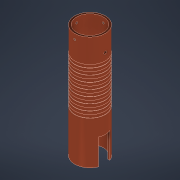
# Autodesk Inventor part: Test_Radiator
Saved by Autodesk Inventor 2022 (Build 260153000, 153)
## iProperties
Created: 2024-05-08
Part Number: Test_Radiator
Material: Generic
Document SubType Name: Modeling
Designer: jo_ki
Density: 1 g/cm^3
Appearance: Copper - Polished
Mass: 36.3453 g
Surface Area: 313.53 cm^2
Volume: 36.3453 cm^3
Author: jo_ki
Autodesk Inventor part; units mm, degrees
note: some values were not read from the file. Chosen so that the rebuilt part matches the saved one: pattern direction of "Circular Pattern1".
ref_plane "XZ Plane" through (0, 0, 0) normal (0, 1, 0) x (-1, 0, 0)
sketch "Sketch1" plane through (0, 0, 0) normal (0, 0, 1) x (1, 0, 0)
  line L0 (0, -89.875) -> (0, 76.375) projected
  line L1 (0, 24.375) -> (14, 24.375)
  line L2 (14, 24.375) -> (14, 21.125)
  line L3 (14, 21.125) -> (20, 21.125)
  line L4 (20, 21.125) -> (20, 17.875)
  line L5 (20, 17.875) -> (14, 17.875)
  line L6 (14, 17.875) -> (14, 14.625)
  line L7 (14, 14.625) -> (20, 14.625)
  line L8 (20, 14.625) -> (20, 11.375)
  line L9 (20, 11.375) -> (14, 11.375)
  line L10 (14, 11.375) -> (14, 8.125)
  line L11 (14, 8.125) -> (20, 8.125)
  line L12 (20, 8.125) -> (20, 4.875)
  line L13 (20, 4.875) -> (14, 4.875)
  line L14 (14, 4.875) -> (14, 1.625)
  line L15 (14, 1.625) -> (20, 1.625)
  line L16 (20, 1.625) -> (20, -1.625)
  line L17 (20, -1.625) -> (14, -1.625)
  line L18 (14, -1.625) -> (14, -4.875)
  line L19 (14, -4.875) -> (20, -4.875)
  line L20 (20, -4.875) -> (20, -8.125)
  line L21 (20, -8.125) -> (14, -8.125)
  line L22 (14, -8.125) -> (14, -11.375)
  line L23 (14, -11.375) -> (20, -11.375)
  line L24 (20, -11.375) -> (20, -14.625)
  line L25 (20, -14.625) -> (14, -14.625)
  line L26 (14, -14.625) -> (14, -17.875)
  line L27 (14, -17.875) -> (20, -17.875)
  line L28 (20, -17.875) -> (20, -21.125)
  line L29 (20, -21.125) -> (14, -21.125)
  line L30 (14, -21.125) -> (14, -24.375)
  line L31 (14, -24.375) -> (0, -24.375)
  line L32 (0, 24.375) -> (0, -24.375)
  line L33 (-4, 0) -> (24, 0) projected
  line L34 (12, 25) -> (12, -24.375)
  line L35 (14, -24.375) -> (14, -34.375)
  line L36 (14, -34.375) -> (12, -34.375)
  line L37 (12, -34.375) -> (12, -24.375)
  line L38 (14, -21.125) -> (16, -21.125)
  line L39 (16, -21.125) -> (16, -66.125)
  line L40 (16, -66.125) -> (14, -66.125)
  line L41 (14, -66.125) -> (14, -21.125)
  line L42 (14, -24.375) -> (14, -24.375)
  line L43 (14, 24.375) -> (20, 24.375)
  line L44 (20, 24.375) -> (20, 27.625)
  line L45 (20, 27.625) -> (14, 27.625)
  line L46 (14, 27.625) -> (14, 52.625)
  line L47 (14, 52.625) -> (12, 52.625)
  line L48 (12, 52.625) -> (12, 25)
  line L49 (12.5, 52.625) -> (12.5, 27.625)
  line L50 (12.5, 27.625) -> (14, 27.625)
  line L51 (12.5, 27.625) -> (12, 27.625)
  line L52 (16, -21.125) -> (16, 52.625)
  line L53 (14, 52.625) -> (16, 52.625)
  line L54 (14, -21.125) -> (14, 52.625)
  line L55 (15.7, -21.125) -> (15.7, 27.625)
  point P0 (14, -34.375)
  point P1 (14, -21.125)
  point P2 (12, 24.375)
  point P3 (12, 25)
  point P4 (16, 21.125)
  point P5 (16, 24.375)
  point P6 (16, 14.625)
  point P7 (16, 17.875)
  point P8 (16, 8.125)
  point P9 (16, 11.375)
  point P10 (16, 1.625)
  point P11 (16, 4.875)
  point P12 (16, -4.875)
  point P13 (16, -1.625)
  point P14 (16, -11.375)
  point P15 (16, -8.125)
  point P16 (16, -17.875)
  point P17 (16, -14.625)
  point P18 (16, 27.625)
  point P19 (15.7, -17.875)
  point P20 (15.7, -14.625)
  point P21 (15.7, -11.375)
  point P22 (15.7, -8.125)
  point P23 (15.7, -4.875)
  point P24 (15.7, -1.625)
  point P25 (15.7, 1.625)
  point P26 (15.7, 4.875)
  point P27 (15.7, 8.125)
  point P28 (15.7, 11.375)
  point P29 (15.7, 14.625)
  point P30 (15.7, 17.875)
  point P31 (15.7, 21.125)
  point P32 (15.7, 24.375)
  point P33 (14, 1.625)
  dimension "d1" = 48.75
  dimension "d3" = 40
  dimension "d4" = 2
  dimension "d6" = 10
  dimension "d12" = 28
  dimension "d13" = 32
  dimension "d15" = 2
  dimension "d25" = 25
  dimension "d37" = 3.25
  dimension "d46" = 1.5
  dimension "d69" = 45
  dimension "d70" = 0.3
  constraints: 108 end point, 37 point on line, 31 perpendicular, 16 equal length, 3 collinear, 3 horizontal, 3 parallel, 1 vertical, 1 other
  measures "d1" distance between parallel lines of L31 L1
  measures "d3" diameter of L28 L0
  measures "d4" distance between parallel lines of L34 L2
  measures "d6" distance of L30.end L35.end
  measures "d12" diameter of L30 L0
  measures "d13" diameter of L39 L0
  measures "d15" distance between parallel lines of L41 L39
  measures "d25" distance between parallel lines of L45 L47
  measures "d37" distance between parallel lines of L27 L29
  measures "d46" distance between parallel lines of L46 L49
  measures "d69" distance between parallel lines of L40 L29
  measures "d70" distance between parallel lines of L55 L52
revolve "Revolution1" add sketch "Sketch1" angle 360 about axis through (0, -10, 0) along (0, 1, 0) contours L30 L29 L39 L40 L41 L35 | L54 L15 L55 L33 | L33 L55 L17 L54 | L54 L27 L55 L29 | L43 L55 L3 L2 | L54 L45 L55 L43 | L17 L55 L19 L18 | L14 L13 L55 L15 | L26 L25 L55 L27 | L3 L55 L5 L54 | L43 L52 L3 L55 | L46 L53 L52 L45 | L17 L52 L19 L55 | L55 L13 L52 L15 | L19 L55 L21 L54 | L54 L11 L55 L13 | L55 L25 L52 L27 | L54 L23 L55 L25 | L5 L55 L7 L6 | L21 L55 L23 L22 | L10 L9 L55 L11 | L5 L52 L7 L55 | L7 L55 L9 L54 | L21 L52 L23 L55 | L55 L9 L52 L11
ref_plane "Work Plane1" through (-16, -43.625, 0) normal (1, 0, 0) x (0, 1, 0)
sketch "Sketch2" plane through (-16, -43.625, 0) normal (1, 0, 0) x (0, 1, 0)
  line L0 (-46.25, 0) -> (120, 0) projected
  line L1 (22.5, 19.8979) -> (22.5, -20.1021)
  line L2 (71.25, 20.5816) -> (71.25, -19.4184)
  line L3 (-22.5, 16) -> (-22.5, -16) projected
  line L4 (96.25, 16) -> (96.25, -16) projected
  line L5 (71.25, 16) -> (71.25, -16) projected
  line L6 (22.5, 16) -> (22.5, -16) projected
  line L7 (-22.5, 16) -> (-22.5, -16) projected
  point P0 (43.625, 0)
  point P1 (-6.5, 0)
  point P2 (-16.5, 0)
  point P3 (90.75, 0)
  point P4 (78.75, 0)
  dimension "d16" = 10
  dimension "d24" = 29
  dimension "d26" = 19.5
  dimension "d58" = 7.5
  constraints: 4 end point, 4 point on line, 2 collinear
  measures "d16" distance of point (-16.5, 0) point (-6.5, 0)
  measures "d24" distance from line of L1 point (-6.5, 0)
  measures "d26" distance from line of L2 point (90.75, 0)
  measures "d58" distance from line of L2 point (78.75, 0)
hole "Hole1" at (-16, -50.125, 0) at (-16, -60.125, 0) direction (1, 0, 0) diameter 2.013 depth 7.6 thread size "M2.5x0.45" class "6H" standard "ISO Metric profile"
hole "Hole2" at (-16, 47.125, 0) direction (1, 0, 0) diameter 2.013 depth 7.6 thread size "M2.5x0.45" class "6H" standard "ISO Metric profile"
pattern_circular "Circular Pattern1" count 3 over 180 about axis through (0, -10, 0) along (0, 1, 0) of "Hole2" both ways yes
ref_plane "Work Plane2" through (16, -43.625, 0) normal (1, 0, 0) x (0, 1, 0)
sketch "Sketch3" plane through (16, -43.625, 0) normal (1, 0, 0) x (0, 1, 0)
  line L0 (-27.5, 6) -> (4.5, 6)
  line L1 (4.5, 6) -> (4.5, -6)
  line L2 (4.5, -6) -> (-27.5, -6)
  line L3 (-27.5, -6) -> (-27.5, 6)
  line L4 (-27.5, 6) -> (4.5, -6) construction
  line L5 (4.5, 6) -> (-27.5, -6) construction
  line L6 (22.5, 21.0012) -> (22.5, -18.9988)
  line L7 (-52.0938, 0) -> (120.974, 0) projected
  line L8 (22.5, 16) -> (22.5, -16) projected
  point P0 (43.625, 0)
  point P1 (-11.5, 0)
  point P2 (-11.5, 0)
  dimension "d41" = 18
  dimension "d42" = 32
  dimension "d43" = 12
  constraints: 14 end point, 3 midpoint, 2 parallel, 1 collinear, 1 horizontal, 1 perpendicular, 1 point on line
  measures "d41" distance between parallel lines of L6 L1
  measures "d42" distance of L1.end L2.end
  measures "d43" distance of L2.end L0.start
extrude "Extrusion1" cut sketch "Sketch3" against normal blind 10
hole "Hole4" at (-16, 35.125, 0) direction (1, 0, 0) diameter 2.9 depth 20 clearance for "Countersunk Flat Head Screw ISO 2009/7046" size "M2.5" standard "ISO"
pattern_circular "Circular Pattern3" count 2 over 360 about axis through (0, -10, 0) along (0, 1, 0) of "Hole4"
body "Solid1"
